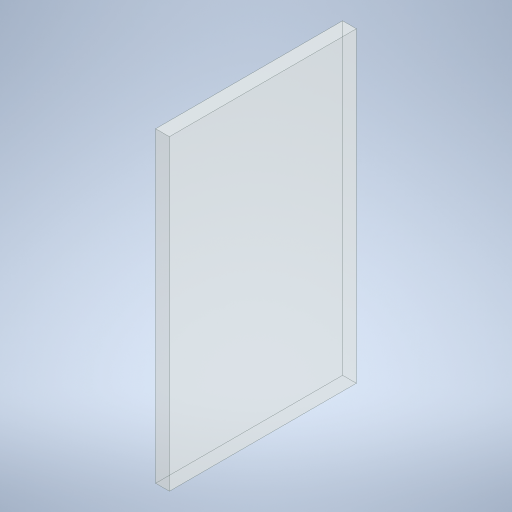
# Autodesk Inventor part: Rear_Wall_For_Existing_Stairwell
Saved by Autodesk Inventor 2024 (Build 280153000, 153)
## iProperties
Created: 2023-05-19
Part Number: Rear_Wall_For_Existing_Stairwell
Material: Wood (Southern Pine)
Document SubType Name: Modeling
Designer: Tom
Density: 7.85 g/cm^3
Appearance: Clear
Author: Tom
Autodesk Inventor part; units mm, degrees
ref_plane "YZ Plane" through (0, 0, 0) normal (1, 0, 0) x (0, 1, 0)
ref_plane "XZ Plane" through (0, 0, 0) normal (0, 1, 0) x (-1, 0, 0)
ref_plane "XY Plane" through (0, 0, 0) normal (0, 0, 1) x (1, 0, 0)
sketch "Sketch1" plane through (0, 0, 0) normal (1, 0, 0) x (0, 1, 0)
  line L0 (0, 0) -> (1981.2, 0)
  line L1 (1981.2, 0) -> (1981.2, -1206.5)
  line L2 (1981.2, -1206.5) -> (0, -1206.5)
  line L3 (0, -1206.5) -> (0, 0)
  dimension "d2" = 1206.5
  dimension "d3" = 1981.2
  constraints: 8 end point, 2 parallel, 1 horizontal, 1 perpendicular
  measures "d2" distance of L2.end L0.start
  measures "d3" distance of L0.start L0.end
extrude "Extrusion1" add sketch "Sketch1" along normal blind 88.9
body "Solid1"
